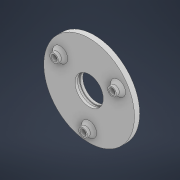
# Autodesk Inventor part: Planet_Carrier_Bottom
Saved by Autodesk Inventor 2021 (Build 250183000, 183)
## iProperties
Created: 2025-03-14
Part Number: Planet_Carrier_Bottom
Material: Generic
Document SubType Name: Modeling
Designer: rocke
Density: 0.558727 g/cm^3
Appearance: Default
Mass: 6.75 g
Surface Area: 57.9116 cm^2
Volume: 12.081 cm^3
3D_PRINTED: True
Author: rocke
Autodesk Inventor part; units mm, degrees
ref_plane "YZ Plane" through (0, 0, 0) normal (1, 0, 0) x (0, 1, 0)
ref_plane "XZ Plane" through (0, 0, 0) normal (0, 1, 0) x (-1, 0, 0)
sketch "Sketch3" plane through (0, 0, 0) normal (0, 0, 1) x (1, 0, 0)
  circle A0 centre (0, 0) radius 26
  dimension "d11" = 52
  constraints: 1 centre point, 1 coincident
  measures "d11" diameter of A0
sketch "Sketch4" plane through (0, 0, 0) normal (0, 0, 1) x (1, 0, 0)
  circle A0 centre (0, -19.155) radius 1.75
  circle A1 centre (0, -19.155) radius 2.5
  circle A2 centre (0, -19.155) radius 5
  circle A3 centre (16.5887, 9.5775) radius 1.75
  circle A4 centre (16.5887, 9.5775) radius 2.5
  circle A5 centre (16.5887, 9.5775) radius 5
  circle A6 centre (-16.5887, 9.5775) radius 1.75
  circle A7 centre (-16.5887, 9.5775) radius 2.5
  circle A8 centre (-16.5887, 9.5775) radius 5
  point P0 (0, 0)
  dimension "d12" = 3.5
  dimension "d13" = 5
  dimension "d14" = 19.155
  dimension "d15" = 10
  dimension "d18" = 360
  constraints: 9 centre point, 6 coincident, 1 vertical alignment, 19 other
  measures "d12" diameter of A0
  measures "d13" diameter of A1
  measures "d14" distance of A0.centre point (0, 0)
  measures "d15" diameter of A2
extrude "Extrusion1" add sketch "Sketch3" against normal blind 3
extrude "Extrusion3" add sketch "Sketch4" along normal blind 3.5 contours A1 | A4 | A7
chamfer "Chamfer1" distance 1.8 angle 45 3 edges at (14.0887, 9.5775, 0) (-19.0887, 9.5775, 0) (-2.5, -19.155, 0)
sketch "Sketch5" plane through (0, 0, -3) normal (0, 0, -1) x (-1, 0, 0)
  circle A0 centre (0, 0) radius 8.1
  dimension "d30" = 16.2
  constraints: 1 centre point, 1 coincident
  measures "d30" diameter of A0
extrude "Extrusion4" cut sketch "Sketch5" against normal up to next
extrude "Extrusion8" cut sketch "Sketch4" against normal through all contours A0 | A3 | A6
sketch "Sketch8" plane through (0, 0, -3) normal (0, 0, -1) x (-1, 0, 0)
  circle A0 centre (0, 0) radius 8.1
  circle A1 centre (0, 0) radius 8.1 projected
  line L0 (10, 5.7735) -> (10, -5.7735)
  line L1 (10, -5.7735) -> (0, -11.547)
  line L2 (0, -11.547) -> (-10, -5.7735)
  line L3 (-10, -5.7735) -> (-10, 5.7735)
  line L4 (-10, 5.7735) -> (0, 11.547)
  line L5 (0, 11.547) -> (10, 5.7735)
  dimension "d46" = 10
  dimension "d53" = 16.2
  constraints: 12 end point, 1 centre point, 1 coincident, 1 vertical alignment, 13 other
  measures "d46" distance from line of point (0, 0) L3
  measures "d53" diameter of A0
extrude "Extrusion10" add sketch "Sketch8" along normal blind 1.5
sketch "Sketch9" plane through (0, 0, 0) normal (0, 0, 1) x (1, 0, 0)
  circle A0 centre (0, 0) radius 8.0468
  circle A1 centre (0, 0) radius 8.6
  dimension "d49" = 17.2
  constraints: 2 centre point, 2 coincident
  measures "d49" diameter of A1
ref_plane "Work Plane2" through (0, 0, -1.5) normal (0, 0, 1) x (1, 0, 0)
extrude "Extrusion11" cut sketch "Sketch9" against normal blind 1.5 from surface at -1.5
body "Solid1"
